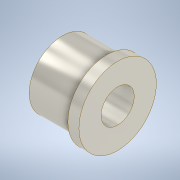
# Autodesk Inventor part: подшипник
Saved by Autodesk Inventor 2020.1 (Build 241239000, 239)
## iProperties
Created: 2021-08-17
Part Number: подшипник
Material: Титан
Document SubType Name: Modeling
Designer: Ni3na
Density: 4.51 g/cm^3
Appearance: Титан
Author: Ni3na
Autodesk Inventor part; units mm, degrees
ref_plane "YZ Plane" through (0, 0, 0) normal (1, 0, 0) x (0, 1, 0)
ref_plane "XZ Plane" through (0, 0, 0) normal (0, 1, 0) x (-1, 0, 0)
ref_plane "XY Plane" through (0, 0, 0) normal (0, 0, 1) x (1, 0, 0)
sketch "Эскиз1" plane through (0, 0, 0) normal (1, 0, 0) x (0, 1, 0)
  circle A0 centre (0, 0) radius 3.5
  circle A1 centre (0, 0) radius 3
  circle A2 centre (0, 0) radius 1.5
  dimension "d0" = 7
  dimension "d1" = 6
  dimension "d2" = 3
  constraints: 3 centre point, 3 coincident
  measures "d0" diameter of A0
  measures "d1" diameter of A1
  measures "d2" diameter of A2
extrude "Выдавливание1" add sketch "Эскиз1" along normal blind 4 contours A1
sketch "Эскиз2" plane through (4, 0, 0) normal (1, 0, 0) x (0, 0, -1)
  circle A0 centre (0, 0) radius 3.5
  circle A1 centre (0, 0) radius 1.5
  dimension "d5" = 7
  constraints: 2 centre point, 2 coincident
  measures "d5" diameter of A0
extrude "Выдавливание2" add sketch "Эскиз2" along normal blind 1
